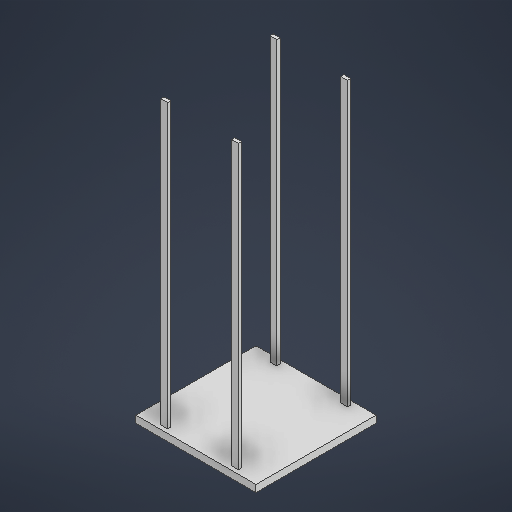
# Autodesk Inventor part: bottom_frame
Saved by Autodesk Inventor 2027 (Build 310192060, 192F)
## iProperties
Created: 2026-07-05
Part Number: bottom_frame
Material: Ogólny
Document SubType Name: Modeling
Designer: User
Density: 1 g/cm^3
Appearance: Domyślna
Author: User
Autodesk Inventor part; units mm, degrees
ref_plane "YZ Plane" through (0, 0, 0) normal (1, 0, 0) x (0, 1, 0)
ref_plane "XZ Plane" through (0, 0, 0) normal (0, 1, 0) x (-1, 0, 0)
ref_plane "XY Plane" through (0, 0, 0) normal (0, 0, 1) x (1, 0, 0)
sketch "Szkic1" plane through (0, 0, 0) normal (0, 1, 0) x (-1, 0, 0)
  line L0 (-17, -17) -> (17, -17)
  line L1 (17, -17) -> (17, 17)
  line L2 (17, 17) -> (-17, 17)
  line L3 (-17, 17) -> (-17, -17)
  line L4 (-17, -17) -> (17, 17) construction
  line L5 (17, -17) -> (-17, 17) construction
  line L6 (-16, -16) -> (16, -16)
  line L7 (16, -16) -> (16, 16)
  line L8 (16, 16) -> (-16, 16)
  line L9 (-16, 16) -> (-16, -16)
  line L10 (-16, -16) -> (16, 16) construction
  line L11 (16, -16) -> (-16, 16) construction
  line L12 (-16, 16) -> (-17, 17)
  line L13 (-16, -16) -> (-17, -17)
  point P0 (0, 0)
  dimension "d0" = 34
  dimension "d1" = 34
  dimension "d2" = 32
  dimension "d3" = 32
  constraints: 28 end point, 4 midpoint, 4 parallel, 2 horizontal, 2 perpendicular
  measures "d0" distance of L2.end L1.end
  measures "d1" distance of L1.end L0.end
  measures "d2" distance of L8.end L7.end
  measures "d3" distance of L7.end L6.end
extrude "Wyciągnięcie proste1" add sketch "Szkic1" against normal blind 2
sketch "Szkic2" plane through (0, 0, 0) normal (0, 1, 0) x (1, 0, 0)
  line L0 (15, 15) -> (-15, 15)
  line L1 (-15, 15) -> (-15, -15)
  line L2 (-15, -15) -> (15, -15)
  line L3 (15, -15) -> (15, 15)
  line L4 (15, 15) -> (-15, -15) construction
  line L5 (-15, 15) -> (15, -15) construction
  line L6 (-15, -15) -> (-11, -15)
  line L7 (-11, -15) -> (-11, -15.9)
  line L8 (-11, -15.9) -> (-9.1, -15.9)
  line L9 (-9.1, -15.9) -> (-9.1, -15)
  line L10 (-9.1, -15.9) -> (-8.2, -15.9) construction
  line L11 (9, -15) -> (9, -15.9)
  line L12 (9, -15.9) -> (10.9, -15.9)
  line L13 (10.9, -15.9) -> (10.9, -15)
  line L14 (10.9, -15.9) -> (11.8, -15.9) construction
  line L15 (-15, 0) -> (15, 0) construction
  line L16 (-11, 15) -> (-11, 15.9)
  line L17 (-11, 15.9) -> (-9.1, 15.9)
  line L18 (-9.1, 15.9) -> (-9.1, 15)
  line L19 (-9.1, 15.9) -> (-8.2, 15.9) construction
  line L20 (9, 15) -> (9, 15.9)
  line L21 (9, 15.9) -> (10.9, 15.9)
  line L22 (10.9, 15.9) -> (10.9, 15)
  line L23 (10.9, 15.9) -> (11.8, 15.9) construction
  point P0 (0, 0)
  dimension "d6" = 30
  dimension "d7" = 30
  dimension "d8" = 4
  dimension "d9" = 0.9
  dimension "d10" = 1.9
  dimension "d12" = 0.9
  dimension "d13" = 90
  dimension "d16" = 20
  constraints: 48 end point, 10 symmetric about line, 5 perpendicular, 4 midpoint, 3 horizontal, 2 parallel, 1 point on line, 9 other
  measures "d6" distance of L2.end L1.end
  measures "d7" distance of L1.end L0.end
  measures "d8" distance of L1.end L6.end
  measures "d9" distance of L6.end L7.end
  measures "d10" distance of L7.end L8.end
  measures "d12" distance of L8.end L9.end
  measures "d13" angle of L10 L9
  measures "d16" distance of L7.end L11.end
extrude "Wyciągnięcie proste2" add sketch "Szkic2" along normal blind 80 contours L0 L20 L21 L22 | L13 L12 L11 L2 | L0 L16 L17 L18 | L9 L8 L7 L2
